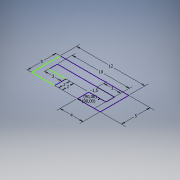
# Autodesk Inventor part: Carro_riel
Saved by Autodesk Inventor 2018 (Build 220112000, 112)
## iProperties
Created: 2021-07-09
Part Number: Carro_riel
Material: Genérico
Document SubType Name: Modeling
Designer: GABRIEL
Density: 1 g/cm^3
Appearance: Valor por defecto
Author: GABRIEL
Autodesk Inventor part; units mm, degrees
ref_plane "YZ Plane" through (0, 0, 0) normal (1, 0, 0) x (0, 1, 0)
ref_plane "XZ Plane" through (0, 0, 0) normal (0, 1, 0) x (-1, 0, 0)
ref_plane "XY Plane" through (0, 0, 0) normal (0, 0, 1) x (1, 0, 0)
sketch "Boceto1" plane through (0, 0, 0) normal (0, 0, 1) x (1, 0, 0)
  line L0 (0, 0) -> (10, 0)
  line L1 (10, 0) -> (10, -1.5)
  line L2 (10, -1.5) -> (7, -1.5)
  line L3 (7, -1.5) -> (7, -3.5)
  line L4 (7, -3.5) -> (3, -3.5)
  line L5 (3, -3.5) -> (3, -1.5)
  line L6 (3, -1.5) -> (0, -1.5)
  line L7 (0, -1.5) -> (0, 0)
  line L8 (-1, 1) -> (11, 1)
  line L9 (11, 1) -> (11, -3.5)
  line L10 (11, -3.5) -> (-1, -3.5)
  line L11 (-1, -3.5) -> (-1, 1)
  dimension "d16" = 10
  dimension "d17" = 1.5
  dimension "d18" = 3
  dimension "d19" = 2
  dimension "d20" = 4
  dimension "d21" = 12
  constraints: 24 end point, 7 perpendicular, 3 point on line, 2 horizontal, 2 parallel
  measures "d16" distance of L0.start L0.end
  measures "d17" distance of L0.end L1.end
  measures "d18" distance of L1.end L2.end
  measures "d19" distance of L2.end L3.end
  measures "d20" distance of L3.end L4.end
  measures "d21" distance of L9.end L10.end
extrude "Extrusión1" add sketch "Boceto1" along normal blind 30 contours L7 L6 L5 L10 L11 L8 L9 L3 L2 L1 L0
